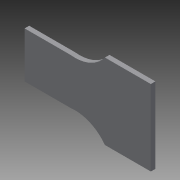
# Autodesk Inventor part: Sweep
Saved by Autodesk Inventor 2014 (Build 180170000, 170)
## iProperties
Created: 2014-03-20
Part Number: Sweep
Material: Generic
Document SubType Name: Modeling
Designer: Pranav
Density: 1 g/cm^3
Appearance: Default
Author: Pranav
Autodesk Inventor part; units mm, degrees
ref_plane "YZ Plane" through (0, 0, 0) normal (1, 0, 0) x (0, 1, 0)
ref_plane "XZ Plane" through (0, 0, 0) normal (0, 1, 0) x (-1, 0, 0)
ref_plane "XY Plane" through (0, 0, 0) normal (0, 0, 1) x (1, 0, 0)
sketch "Sketch1" plane through (0, 0, 0) normal (0, 0, 1) x (1, 0, 0)
  line L0 (-25.4, 0) -> (-25.4, -12.7)
  line L1 (19.05, 8.255) -> (44.45, 8.255)
  line L2 (44.45, 8.255) -> (44.45, -12.7)
  line L3 (0, -25.4) -> (-25.4, -25.4)
  line L4 (-25.4, -25.4) -> (-25.4, -12.7)
  line L5 (19.05, -33.655) -> (44.45, -33.655)
  line L6 (44.45, -33.655) -> (44.45, -12.7)
  line L7 (-25.4, 0) -> (0, 0)
  arc A0 (0, 0) -> (19.05, 8.255) centre (2.4365, 20.4857) ccw
  arc A1 (19.05, -33.655) -> (0, -25.4) centre (2.4389, -45.8801) ccw
  dimension "d2" = 12.7
  dimension "d3" = 25.4
  dimension "d4" = 20.955
  dimension "d5" = 20.955
  dimension "d6" = 20.6248
  constraints: 16 end point, 4 point on circle, 2 centre point, 2 perpendicular
  measures "d2" distance of L0.start L0.end
  measures "d3" distance of L1.start L1.end
  measures "d4" distance of L1.end L2.end
  measures "d5" distance of L5.end L2.end
  measures "d6" radius of A1
extrude "Extrusion1" add sketch "Sketch1" along normal blind 2.54
body "Solid1"
